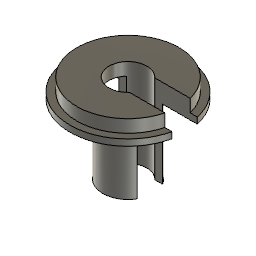
tube_adapter_centrifuge_50ml (Autodesk Fusion 360 design; units mm, degrees)
Autodesk Fusion 360 part; units mm, degrees
note: some values were not read from the file. Set by a fixed rule: which sketch regions a step uses.
sketch "スケッチ1" plane through (0, 0, 0) normal (0, 0, 1) x (1, 0, 0)
  circle A0 centre (0, 0) radius 46
  dimension "d1" = 92
  constraint coincident A0.centre origin
  measures "d1" diameter of A0
extrude "押し出し1" add sketch "スケッチ1" along normal blind 70
sketch "スケッチ2" plane through (0, 0, 70) normal (0, 0, 1) x (-1, 0, 0)
  circle A0 centre (0, 0) radius 46
  circle A1 centre (0, 0) radius 40.5
  dimension "d4" = 81
  constraint coincident A0.centre A1.centre
  measures "d4" diameter of A1
extrude "押し出し2" cut sketch "スケッチ2" against normal blind 10
sketch "スケッチ3" plane through (0, 0, 70) normal (0, 0, 1) x (-1, 0, 0)
  circle A0 centre (0, 0) radius 40.5
  circle A1 centre (0, 0) radius 15
  dimension "d7" = 30
  constraint coincident A0.centre A1.centre
  measures "d7" diameter of A1
extrude "押し出し3" cut sketch "スケッチ3" against normal blind 100 contours A1
sketch "スケッチ4" plane through (0, 0, 0) normal (0, 0, -1) x (1, 0, 0)
  circle A0 centre (0, 0) radius 15
  circle A1 centre (0, 0) radius 46
  circle A2 centre (0, 0) radius 20
  dimension "d12" = 40
  constraint concentric A0 A2
  measures "d12" diameter of A2
extrude "押し出し4" cut sketch "スケッチ4" against normal blind 55 contours A1
sketch "スケッチ5" plane through (0, 0, 0) normal (0, 0, -1) x (1, 0, 0)
  circle A0 centre (0, 0) radius 20
  circle A1 centre (0, 0) radius 15
  line L0 (-55, 10) -> (55, 10)
  line L1 (55, 10) -> (55, -10)
  line L2 (55, -10) -> (-55, -10)
  line L3 (-55, -10) -> (-55, 10)
  constraint horizontal L0
  constraint vertical L1
  constraint horizontal L2
  constraint vertical L3
extrude "押し出し5" cut sketch "スケッチ5" against normal blind 60 contours A0 A1 L0 L2 | A0 L0 L1 L2 | A0 A1 L0 L2 | A0 L0 L2 L3
extrude "押し出し6" cut 1 faces at (31.4239, 5.7402, 60) along direction (0, 0, 1) blind 10
fillet "フィレット1" [suppressed]
